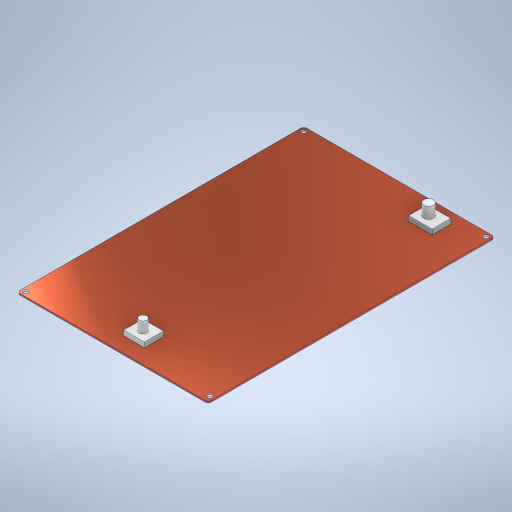
# Autodesk Inventor part: PCB
Saved by Autodesk Inventor 2023 (Build 270158000, 158)
## iProperties
Created: 2023-03-21
Part Number: PCB
Material: Aluminum 6061
Document SubType Name: Sheet Metal
Designer: Inteli
Density: 2.7 g/cm^3
Sheet Metal Rule: Default
Appearance: Aluminum - Flat
Author: Inteli
Autodesk Inventor part; units mm, degrees
ref_plane "YZ Plane" through (0, 0, 0) normal (1, 0, 0) x (0, 1, 0)
ref_plane "XZ Plane" through (0, 0, 0) normal (0, 1, 0) x (-1, 0, 0)
ref_plane "XY Plane" through (0, 0, 0) normal (0, 0, 1) x (1, 0, 0)
sketch "Sketch1" plane through (0, 0, 0) normal (0, 1, 0) x (-1, 0, 0)
  line L0 (0, 0) -> (0, -180)
  line L1 (0, -180) -> (-120, -180)
  line L2 (-120, -180) -> (-120, 0)
  line L3 (-120, 0) -> (0, 0)
  dimension "d1" = 180
  dimension "d2" = 120
  constraints: 8 end point, 3 perpendicular, 1 vertical
  measures "d1" distance of L0.start L0.end
  measures "d2" distance of L0.end L1.end
extrude "Extrusion1" add sketch "Sketch1" along normal blind 1
fillet "Fillet1" radius 2 4 edges at (0, 0.5, 0) (120, 0.5, 0) (120, 0.5, -180) (0, 0.5, -180)
sketch "Sketch2" plane through (0, 1, 0) normal (0, 1, 0) x (1, 0, 0)
  arc A0 (2, 180) -> (0, 178) centre (2, 178) ccw projected
  circle A1 centre (2.7071, 177.2929) radius 1.5
  line L0 (2, 0) -> (118, 0) projected
  line L1 (118, 180) -> (2, 180) projected
  arc A2 (120, 178) -> (118, 180) centre (118, 178) ccw projected
  circle A3 centre (117.2929, 177.2929) radius 1.5
  arc A4 (118, 0) -> (120, 2) centre (118, 2) ccw projected
  circle A5 centre (117.2929, 3.7977) radius 1.5
  arc A6 (0, 2) -> (2, 0) centre (2, 2) ccw projected
  circle A7 centre (2.7071, 2.7071) radius 1.5
  point P0 (0, 0)
  dimension "d7" = 3
  dimension "d10" = 3
  dimension "d11" = 3
  constraints: 4 centre point
  measures "d7" diameter of A1
  measures "d10" diameter of A3
  measures "d11" diameter of A5
extrude "Extrusion2" cut sketch "Sketch2" against normal through all
sketch "Sketch3" plane through (0, 1, 0) normal (0, 1, 0) x (1, 0, 0)
  line L0 (57.2525, 21.6143) -> (70.3337, 21.6143)
  line L1 (70.3337, 21.6143) -> (70.3337, 9.5938)
  line L2 (70.3337, 9.5938) -> (57.2525, 9.5938)
  line L3 (57.2525, 9.5938) -> (57.2525, 21.6143)
  line L4 (84.4572, 173.1647) -> (99.2564, 173.1647)
  line L5 (99.2564, 173.1647) -> (99.2564, 161.3857)
  line L6 (99.2564, 161.3857) -> (84.4572, 161.3857)
  line L7 (84.4572, 161.3857) -> (84.4572, 173.1647)
  point P0 (0, 0)
  constraints: 16 end point, 4 parallel, 2 horizontal, 2 perpendicular
extrude "Extrusion3" add sketch "Sketch3" along normal blind 10
sketch "Sketch4" plane through (0, 11, 0) normal (0, 1, 0) x (1, 0, 0)
  circle A0 centre (63.7549, 15.2444) radius 2.3335
  circle A1 centre (90.6401, 167.8396) radius 3.0183
  line L0 (57.2525, 9.5938) -> (70.3337, 9.5938) projected
  line L1 (70.3337, 21.6143) -> (70.3337, 9.5938)
  line L2 (70.3337, 9.5938) -> (57.2525, 9.5938)
  line L3 (57.2525, 9.5938) -> (57.2525, 21.6143)
  line L4 (57.2525, 21.6143) -> (70.3337, 21.6143)
  line L5 (99.2564, 161.3857) -> (99.2564, 173.1647) projected
  line L6 (84.4572, 173.1647) -> (99.2564, 173.1647)
  line L7 (99.2564, 173.1647) -> (99.2564, 161.3857)
  line L8 (99.2564, 161.3857) -> (84.4572, 161.3857)
  line L9 (84.4572, 173.1647) -> (84.4572, 161.3857) projected
  line L10 (84.4572, 161.3857) -> (84.4572, 173.1647)
  point P0 (0, 0)
  constraints: 16 end point, 3 collinear, 3 perpendicular, 2 centre point, 1 horizontal, 1 vertical
extrude "Extrusion4" cut sketch "Sketch4" against normal blind 7
equation "\"BendRadius\" = Thickness"
equation "\"BendReliefWidth\" = Thickness"
equation "\"BendReliefDepth\" = 0.5 * Thickness"
equation "\"CornerReliefSize\" = 4 * Thickness"
equation "\"MinimumRemnant\" = 2 * Thickness"
equation "\"TransitionRadius\" = BendRadius"
equation "\"JacobiRadiusSize\" = BendRadius"
equation "\"GapSize\" = Thickness"
equation "\"Thickness\" = 3.048"
body "Solid1"
